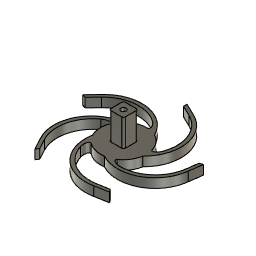
Ratchet v3 (Autodesk Fusion 360 design; units mm, degrees)
Autodesk Fusion 360 part; units mm, degrees
sketch "bottom" plane through (0, 0, 0) normal (0, 0, 1) x (1, 0, 0)
  circle A0 centre (0, 0) radius 2.25
  line L0 (4.15, 0) -> (2.075, 3.594)
  line L1 (2.075, 3.594) -> (-2.075, 3.594)
  line L2 (-2.075, 3.594) -> (-4.15, 0)
  line L3 (-4.15, 0) -> (-2.075, -3.594)
  line L4 (-2.075, -3.594) -> (2.075, -3.594)
  line L5 (2.075, -3.594) -> (4.15, 0)
  line L6 (4.75, 6.25) -> (-4.75, 6.25)
  line L7 (-6.25, 4.75) -> (-6.25, -4.75)
  line L8 (-4.75, -6.25) -> (4.75, -6.25)
  line L9 (6.25, -4.75) -> (6.25, 4.75)
  line L10 (6.25, 6.25) -> (-6.25, -6.25) construction
  line L11 (-6.25, 6.25) -> (6.25, -6.25) construction
  arc A1 (4.75, -6.25) -> (6.25, -4.75) centre (4.75, -4.75) ccw
  arc A2 (-6.25, -4.75) -> (-4.75, -6.25) centre (-4.75, -4.75) ccw
  arc A3 (-4.75, 6.25) -> (-6.25, 4.75) centre (-4.75, 4.75) ccw
  arc A4 (6.25, 4.75) -> (4.75, 6.25) centre (4.75, 4.75) ccw
  circle A5 centre (0, 0) radius 20
  circle A6 centre (0, 0) radius 55
  line L12 (0, 55) -> (0, 52)
  line L13 (0, 55) -> (10.5968, 49.8773)
  line L14 (0, 55) -> (11.77, 55) construction
  line L15 (0, 52) -> (10.5968, 46.8773)
  arc A7 (25.1153, 10.0637) -> (9.1347, 47.5841) centre (-4.3574, 19.6742) ccw
  arc A8 (19.7662, -3.0491) -> (10.5968, 49.8773) centre (-2.8509, 20.29) ccw
  spline S0 degree 5 poles (19.2844, 5.302) (19.288, 5.2968) (19.3924, 5.1455) (19.6116, 4.8896) (19.9793, 4.632) (20.5483, 4.5429) (21.3688, 4.8461) (22.2615, 5.515) (23.1597, 6.4634) (23.9893, 7.5946) (24.5403, 8.5729) (24.8652, 9.3175) (25.039, 9.8148) (25.1153, 10.0637) knots 0.196493 0.196493 0.196493 0.196493 0.196493 0.196493 0.2 0.3 0.4 0.5 0.6 0.7 0.8 0.9 1 1 1 1 1 1
  line L16 (18.6573, 6.2172) -> (19.9116, 4.3867)
  line L17 (24.8256, 9.1182) -> (25.4049, 11.0092)
  point P0 (20.8497, 4.7036)
  dimension "d1" = 4.5
  dimension "d2" = 4.15
  dimension "d3" = 12.5
  dimension "d4" = 12.5
  dimension "d5" = 1.5
  dimension "d6" = 1.5
  dimension "d7" = 1.5
  dimension "d8" = 40
  dimension "d9" = 110
  dimension "d10" = 3
  dimension "d11" = 25.8
  dimension "d12" = 11.77
  dimension "d13" = 11.77
  dimension "d14" = 62
  dimension "d16" = 65
  constraint coincident A0.centre A5.centre
  constraint horizontal L6
  constraint perpendicular L6 L7
  constraint parallel L6 L8
  constraint parallel L7 L9
  constraint coincident L10 A0.centre
  constraint coincident L11 A0.centre
  constraint coincident L11.end L8
  constraint coincident L11.end L9
  constraint tangent L8 A1
  constraint tangent L9 A1
  constraint coincident L10.end L8
  constraint coincident L10.end L7
  constraint tangent L8 A2
  constraint tangent L7 A2
  constraint coincident L11.start L7
  constraint coincident L11.start L6
  constraint tangent L7 A3
  constraint tangent L6 A3
  constraint equal A2 A3
  constraint coincident L10.start L6
  constraint coincident L10.start L9
  constraint tangent L6 A4
  constraint tangent L9 A4
  constraint coincident A6 L12.start
  constraint vertical L12
  constraint horizontal L14
  constraint tangent L15 A7
  constraint coincident L15 A7.end
  constraint coincident A5 A8.start
  constraint coincident A5 S0.start
  constraint midpoint S0.start L16
  constraint midpoint A7.start L17
  measures "d1" diameter of A0
  measures "d2" distance of L0.start A0.centre
  measures "d3" distance of L10.end L11.end
  measures "d4" distance of L11.start L10.end
  measures "d5" radius of A1
  measures "d6" radius of A2
  measures "d7" radius of A4
  measures "d8" diameter of A5
  measures "d9" diameter of A6
  measures "d10" distance of L12.start L12.end
  measures "d11" angle of L13 L14
  measures "d12" distance of L12.start L13.end
  measures "d13" distance of L12.end L15.end
  measures "d14" diameter of A7
  measures "d16" diameter of A8
extrude "Extrude2" add sketch "bottom" along normal blind 8 contours A5 L12 L13 L15 A7 A8 S0 L17 makes body 1
pattern_circular "C-Pattern1" count 5 over 360 about axis through (0, 0, 0) along (0, 0, 1) of "Extrude2" makes body 2 makes body 3 makes body 4 makes body 5
extrude "Extrude3" add sketch "bottom" along normal blind 8 contours L0 L1 L2 L3 L4 L5 | L6 L7 L8 L9 A1 A2 A3 A4 | A5 bodies 1 2 3 4 5
extrude "Extrude4" add sketch "bottom" along normal blind 31.5 contours L0 L1 L2 L3 L4 L5 | L6 L7 L8 L9 A1 A2 A3 A4 bodies 1
extrude "Extrude5" cut sketch "bottom" along normal blind 4 contours L0 L1 L2 L3 L4 L5 bodies 1
equation "d2 = ( 8.3 / 2 ) * 1 mm"
equation "d11 = 90 deg - 64.2 deg"
named bodies: "Ratchet"
